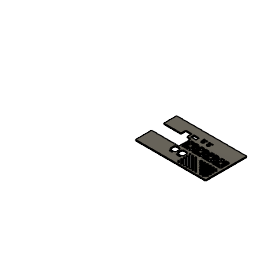
HomecurrentMoniter_Top Plate HCM UPDATED (Autodesk Fusion 360 design; units mm, degrees)
part number: 2026-06-16-14-02-59-231
Autodesk Fusion 360 part; units mm, degrees
(part 1 of 5)
sketch "Sketch1" plane through (0, 0, 20) normal (0, 0, 1) x (-1, 0, 0)
  line L0 (-199.377, 36.7921) -> (-199.377, 118.6521)
  line L1 (-199.377, 118.6521) -> (-338.527, 118.6521)
  line L2 (-338.527, 118.6521) -> (-338.527, 36.7921)
  line L3 (-338.527, 36.7921) -> (-199.377, 36.7921)
  line L4 (-257.2248, 89.2793) -> (-251.8248, 89.2793)
  arc A0 (-251.8248, 89.2793) -> (-248.7748, 92.3293) centre (-251.8248, 92.3293) ccw
  line L5 (-248.7748, 92.3293) -> (-248.7748, 97.7293)
  arc A1 (-248.7748, 97.7293) -> (-251.8248, 100.7793) centre (-251.8248, 97.7293) ccw
  line L6 (-251.8248, 100.7793) -> (-257.2248, 100.7793)
  arc A2 (-257.2248, 100.7793) -> (-260.2748, 97.7293) centre (-257.2248, 97.7293) ccw
  line L7 (-260.2748, 97.7293) -> (-260.2748, 92.3293)
  arc A3 (-260.2748, 92.3293) -> (-257.2248, 89.2793) centre (-257.2248, 92.3293) ccw
  line L8 (-271.6198, 89.1213) -> (-266.2198, 89.1213)
  arc A4 (-266.2198, 89.1213) -> (-263.1698, 92.1713) centre (-266.2198, 92.1713) ccw
  arc A5 (-274.6698, 92.1713) -> (-271.6198, 89.1213) centre (-271.6198, 92.1713) ccw
  line L9 (-274.6698, 97.5713) -> (-274.6698, 92.1713)
  arc A6 (-271.6198, 100.6213) -> (-274.6698, 97.5713) centre (-271.6198, 97.5713) ccw
  line L10 (-266.2198, 100.6213) -> (-271.6198, 100.6213)
  arc A7 (-263.1698, 97.5713) -> (-266.2198, 100.6213) centre (-266.2198, 97.5713) ccw
  line L11 (-263.1698, 92.1713) -> (-263.1698, 97.5713)
  arc A8 (-268.8911, 56.8718) -> (-268.8911, 54.5394) centre (-270.3911, 55.7056) ccw
  line L12 (-268.8911, 56.8718) -> (-268.8911, 54.5394)
  arc A9 (-280.0411, 56.9618) -> (-280.0411, 54.6294) centre (-281.5411, 55.7956) ccw
  line L13 (-280.0411, 56.9618) -> (-280.0411, 54.6294)
  line L14 (-251.0886, 55.7428) -> (-251.3426, 55.9968)
  line L15 (-251.3426, 55.9968) -> (-253.3746, 55.9968)
  line L16 (-253.3746, 55.9968) -> (-253.6286, 55.7428)
  line L17 (-253.6286, 55.7428) -> (-253.8826, 55.9968)
  line L18 (-253.8826, 55.9968) -> (-255.9146, 55.9968)
  line L19 (-255.9146, 55.9968) -> (-256.1686, 55.7428)
  line L20 (-256.1686, 55.7428) -> (-256.4226, 55.9968)
  line L21 (-256.4226, 55.9968) -> (-258.4546, 55.9968)
  line L22 (-258.4546, 55.9968) -> (-258.7086, 55.7428)
  line L23 (-258.7086, 55.7428) -> (-258.7086, 53.7108)
  line L24 (-258.7086, 53.7108) -> (-258.4546, 53.4568)
  line L25 (-258.4546, 53.4568) -> (-256.4226, 53.4568)
  line L26 (-256.4226, 53.4568) -> (-256.1686, 53.7108)
  line L27 (-256.1686, 53.7108) -> (-255.9146, 53.4568)
  line L28 (-255.9146, 53.4568) -> (-253.8826, 53.4568)
  line L29 (-253.8826, 53.4568) -> (-253.6286, 53.7108)
  line L30 (-253.6286, 53.7108) -> (-253.3746, 53.4568)
  line L31 (-253.3746, 53.4568) -> (-251.3426, 53.4568)
  line L32 (-251.3426, 53.4568) -> (-251.0886, 53.7108)
  line L33 (-251.0886, 53.7108) -> (-251.0886, 55.7428)
  line L34 (-234.5786, 55.7428) -> (-234.8326, 55.9968)
  line L35 (-234.8326, 55.9968) -> (-236.8646, 55.9968)
  line L36 (-236.8646, 55.9968) -> (-237.1186, 55.7428)
  line L37 (-237.1186, 55.7428) -> (-237.3726, 55.9968)
  line L38 (-237.3726, 55.9968) -> (-239.4046, 55.9968)
  line L39 (-239.4046, 55.9968) -> (-239.6586, 55.7428)
  line L40 (-239.6586, 55.7428) -> (-239.9126, 55.9968)
  line L41 (-239.9126, 55.9968) -> (-241.9446, 55.9968)
  line L42 (-241.9446, 55.9968) -> (-242.1986, 55.7428)
  line L43 (-242.1986, 55.7428) -> (-242.4526, 55.9968)
  line L44 (-242.4526, 55.9968) -> (-244.4846, 55.9968)
  line L45 (-244.4846, 55.9968) -> (-244.7386, 55.7428)
  line L46 (-244.7386, 55.7428) -> (-244.7386, 53.7108)
  line L47 (-244.7386, 53.7108) -> (-244.4846, 53.4568)
  line L48 (-244.4846, 53.4568) -> (-242.4526, 53.4568)
  line L49 (-242.4526, 53.4568) -> (-242.1986, 53.7108)
  line L50 (-242.1986, 53.7108) -> (-241.9446, 53.4568)
  line L51 (-241.9446, 53.4568) -> (-239.9126, 53.4568)
  line L52 (-239.9126, 53.4568) -> (-239.6586, 53.7108)
  line L53 (-239.6586, 53.7108) -> (-239.4046, 53.4568)
  line L54 (-239.4046, 53.4568) -> (-237.3726, 53.4568)
  line L55 (-237.3726, 53.4568) -> (-237.1186, 53.7108)
  line L56 (-237.1186, 53.7108) -> (-236.8646, 53.4568)
  line L57 (-236.8646, 53.4568) -> (-234.8326, 53.4568)
  line L58 (-234.8326, 53.4568) -> (-234.5786, 53.7108)
  line L59 (-234.5786, 53.7108) -> (-234.5786, 55.7428)
  line L60 (-249.9009, 53) -> (-259.9009, 53)
  line L61 (-259.9009, 53) -> (-259.9009, 59)
  line L62 (-259.9009, 59) -> (-249.9009, 59)
  line L63 (-249.9009, 59) -> (-249.9009, 53)
  line L64 (-233.633, 53) -> (-245.633, 53)
  line L65 (-245.633, 53) -> (-245.633, 75)
  line L66 (-245.633, 75) -> (-233.633, 75)
  line L67 (-233.633, 75) -> (-233.633, 53)
  circle A10 centre (-270.3911, 55.7056) radius 3
  circle A11 centre (-281.5411, 55.7956) radius 3
  line L68 (-232.1048, 83.5518) -> (-224.9198, 83.5518)
  line L69 (-224.9198, 83.5518) -> (-224.9198, 65.5518)
  line L70 (-224.9198, 65.5518) -> (-232.1048, 65.5518)
  line L71 (-232.1098, 65.5518) -> (-232.1048, 65.5518)
  line L72 (-232.2048, 65.5518) -> (-232.1098, 65.5518)
  arc A12 (-232.2048, 65.5518) -> (-232.7048, 65.5518) centre (-232.4548, 65.5518) ccw
  line L73 (-232.7098, 65.5518) -> (-232.7048, 65.5518)
  line L74 (-232.8048, 65.5518) -> (-232.7098, 65.5518)
  line L75 (-232.8048, 65.5518) -> (-233.3748, 65.5518)
  line L76 (-233.3798, 65.5518) -> (-233.3748, 65.5518)
  line L77 (-233.4748, 65.5518) -> (-233.3798, 65.5518)
  arc A13 (-233.4748, 65.5518) -> (-233.9748, 65.5518) centre (-233.7248, 65.5518) ccw
  line L78 (-233.9798, 65.5518) -> (-233.9748, 65.5518)
  line L79 (-234.0748, 65.5518) -> (-233.9798, 65.5518)
  line L80 (-234.0748, 65.5518) -> (-234.6448, 65.5518)
  line L81 (-234.6498, 65.5518) -> (-234.6448, 65.5518)
  line L82 (-234.7448, 65.5518) -> (-234.6498, 65.5518)
  arc A14 (-234.7448, 65.5518) -> (-235.2448, 65.5518) centre (-234.9948, 65.5518) ccw
  line L83 (-235.2498, 65.5518) -> (-235.2448, 65.5518)
  line L84 (-235.3448, 65.5518) -> (-235.2498, 65.5518)
  line L85 (-235.3448, 65.5518) -> (-235.9148, 65.5518)
  line L86 (-235.9198, 65.5518) -> (-235.9148, 65.5518)
  line L87 (-236.0148, 65.5518) -> (-235.9198, 65.5518)
  arc A15 (-236.0148, 65.5518) -> (-236.5148, 65.5518) centre (-236.2648, 65.5518) ccw
  line L88 (-236.5198, 65.5518) -> (-236.5148, 65.5518)
  line L89 (-236.6148, 65.5518) -> (-236.5198, 65.5518)
  line L90 (-236.6148, 65.5518) -> (-237.1848, 65.5518)
  line L91 (-237.1898, 65.5518) -> (-237.1848, 65.5518)
  line L92 (-237.2848, 65.5518) -> (-237.1898, 65.5518)
  arc A16 (-237.2848, 65.5518) -> (-237.7848, 65.5518) centre (-237.5348, 65.5518) ccw
  line L93 (-237.7898, 65.5518) -> (-237.7848, 65.5518)
  line L94 (-237.8848, 65.5518) -> (-237.7898, 65.5518)
  line L95 (-237.8848, 65.5518) -> (-238.4548, 65.5518)
  line L96 (-238.4598, 65.5518) -> (-238.4548, 65.5518)
  line L97 (-238.5548, 65.5518) -> (-238.4598, 65.5518)
  arc A17 (-238.5548, 65.5518) -> (-239.0548, 65.5518) centre (-238.8048, 65.5518) ccw
  line L98 (-239.0598, 65.5518) -> (-239.0548, 65.5518)
  line L99 (-239.1548, 65.5518) -> (-239.0598, 65.5518)
  line L100 (-239.1548, 65.5518) -> (-239.7248, 65.5518)
  line L101 (-239.7298, 65.5518) -> (-239.7248, 65.5518)
  line L102 (-239.8248, 65.5518) -> (-239.7298, 65.5518)
  arc A18 (-239.8248, 65.5518) -> (-240.3248, 65.5518) centre (-240.0748, 65.5518) ccw
  line L103 (-240.3298, 65.5518) -> (-240.3248, 65.5518)
  line L104 (-240.4248, 65.5518) -> (-240.3298, 65.5518)
  line L105 (-240.4248, 65.5518) -> (-240.9948, 65.5518)
  line L106 (-240.9998, 65.5518) -> (-240.9948, 65.5518)
  line L107 (-241.0948, 65.5518) -> (-240.9998, 65.5518)
  arc A19 (-241.0948, 65.5518) -> (-241.5948, 65.5518) centre (-241.3448, 65.5518) ccw
  line L108 (-241.5998, 65.5518) -> (-241.5948, 65.5518)
  line L109 (-241.6948, 65.5518) -> (-241.5998, 65.5518)
  line L110 (-241.6948, 65.5518) -> (-242.2648, 65.5518)
  line L111 (-242.2698, 65.5518) -> (-242.2648, 65.5518)
  line L112 (-242.3648, 65.5518) -> (-242.2698, 65.5518)
  arc A20 (-242.3648, 65.5518) -> (-242.8648, 65.5518) centre (-242.6148, 65.5518) ccw
  line L113 (-242.8698, 65.5518) -> (-242.8648, 65.5518)
  line L114 (-242.9648, 65.5518) -> (-242.8698, 65.5518)
  line L115 (-242.9648, 65.5518) -> (-243.5348, 65.5518)
  line L116 (-243.5398, 65.5518) -> (-243.5348, 65.5518)
  line L117 (-243.6348, 65.5518) -> (-243.5398, 65.5518)
  arc A21 (-243.6348, 65.5518) -> (-244.1348, 65.5518) centre (-243.8848, 65.5518) ccw
  line L118 (-244.1398, 65.5518) -> (-244.1348, 65.5518)
  line L119 (-244.2348, 65.5518) -> (-244.1398, 65.5518)
  line L120 (-244.2348, 65.5518) -> (-244.8048, 65.5518)
  line L121 (-244.8098, 65.5518) -> (-244.8048, 65.5518)
  line L122 (-244.9048, 65.5518) -> (-244.8098, 65.5518)
  arc A22 (-244.9048, 65.5518) -> (-245.4048, 65.5518) centre (-245.1548, 65.5518) ccw
  line L123 (-245.4098, 65.5518) -> (-245.4048, 65.5518)
  line L124 (-245.5048, 65.5518) -> (-245.4098, 65.5518)
  line L125 (-245.5048, 65.5518) -> (-246.0748, 65.5518)
  line L126 (-246.0798, 65.5518) -> (-246.0748, 65.5518)
  line L127 (-246.1748, 65.5518) -> (-246.0798, 65.5518)
  arc A23 (-246.1748, 65.5518) -> (-246.6748, 65.5518) centre (-246.4248, 65.5518) ccw
  line L128 (-246.6798, 65.5518) -> (-246.6748, 65.5518)
  line L129 (-246.7748, 65.5518) -> (-246.6798, 65.5518)
  line L130 (-246.7748, 65.5518) -> (-247.3448, 65.5518)
  line L131 (-247.3498, 65.5518) -> (-247.3448, 65.5518)
  line L132 (-247.4448, 65.5518) -> (-247.3498, 65.5518)
  arc A24 (-247.4448, 65.5518) -> (-247.9448, 65.5518) centre (-247.6948, 65.5518) ccw
  line L133 (-247.9498, 65.5518) -> (-247.9448, 65.5518)
  line L134 (-248.0448, 65.5518) -> (-247.9498, 65.5518)
  line L135 (-248.0448, 65.5518) -> (-248.6148, 65.5518)
  line L136 (-248.6198, 65.5518) -> (-248.6148, 65.5518)
  line L137 (-248.7148, 65.5518) -> (-248.6198, 65.5518)
  arc A25 (-248.7148, 65.5518) -> (-249.2148, 65.5518) centre (-248.9648, 65.5518) ccw
  line L138 (-249.2198, 65.5518) -> (-249.2148, 65.5518)
  line L139 (-249.3148, 65.5518) -> (-249.2198, 65.5518)
  line L140 (-249.3148, 65.5518) -> (-250.4198, 65.5518)
  line L141 (-250.4198, 65.5518) -> (-250.4198, 68.4418)
  line L142 (-250.4198, 68.5369) -> (-250.4198, 68.4418)
  line L143 (-250.4198, 68.5418) -> (-250.4198, 68.5369)
  arc A26 (-250.4198, 68.5418) -> (-250.4198, 69.0418) centre (-250.4198, 68.7918) ccw
  line L144 (-250.4198, 69.1368) -> (-250.4198, 69.0418)
  line L145 (-250.4198, 69.1418) -> (-250.4198, 69.1368)
  line L146 (-250.4198, 69.1418) -> (-250.4198, 69.7118)
  line L147 (-250.4198, 69.8069) -> (-250.4198, 69.7118)
  line L148 (-250.4198, 69.8118) -> (-250.4198, 69.8069)
  arc A27 (-250.4198, 69.8118) -> (-250.4198, 70.3118) centre (-250.4198, 70.0618) ccw
  line L149 (-250.4198, 70.4068) -> (-250.4198, 70.3118)
  line L150 (-250.4198, 70.4118) -> (-250.4198, 70.4068)
  line L151 (-250.4198, 70.4118) -> (-250.4198, 70.9818)
  line L152 (-250.4198, 71.0769) -> (-250.4198, 70.9818)
  line L153 (-250.4198, 71.0818) -> (-250.4198, 71.0769)
  arc A28 (-250.4198, 71.0818) -> (-250.4198, 71.5818) centre (-250.4198, 71.3318) ccw
  line L154 (-250.4198, 71.6768) -> (-250.4198, 71.5818)
  line L155 (-250.4198, 71.6818) -> (-250.4198, 71.6768)
  line L156 (-250.4198, 71.6818) -> (-250.4198, 72.2518)
  line L157 (-250.4198, 72.3469) -> (-250.4198, 72.2518)
  line L158 (-250.4198, 72.3518) -> (-250.4198, 72.3469)
  arc A29 (-250.4198, 72.3518) -> (-250.4198, 72.8518) centre (-250.4198, 72.6018) ccw
  line L159 (-250.4198, 72.9468) -> (-250.4198, 72.8518)
  line L160 (-250.4198, 72.9518) -> (-250.4198, 72.9468)
  line L161 (-250.4198, 72.9518) -> (-250.4198, 73.5218)
  line L162 (-250.4198, 73.6169) -> (-250.4198, 73.5218)
  line L163 (-250.4198, 73.6218) -> (-250.4198, 73.6169)
  arc A30 (-250.4198, 73.6218) -> (-250.4198, 74.1218) centre (-250.4198, 73.8718) ccw
  line L164 (-250.4198, 74.2168) -> (-250.4198, 74.1218)
  line L165 (-250.4198, 74.2218) -> (-250.4198, 74.2168)
  line L166 (-250.4198, 74.2218) -> (-250.4198, 74.7918)
  line L167 (-250.4198, 74.8869) -> (-250.4198, 74.7918)
  line L168 (-250.4198, 74.8918) -> (-250.4198, 74.8869)
  arc A31 (-250.4198, 74.8918) -> (-250.4198, 75.3918) centre (-250.4198, 75.1418) ccw
  line L169 (-250.4198, 75.4868) -> (-250.4198, 75.3918)
  line L170 (-250.4198, 75.4918) -> (-250.4198, 75.4868)
  line L171 (-250.4198, 75.4918) -> (-250.4198, 76.0618)
  line L172 (-250.4198, 76.1569) -> (-250.4198, 76.0618)
  line L173 (-250.4198, 76.1618) -> (-250.4198, 76.1569)
  arc A32 (-250.4198, 76.1618) -> (-250.4198, 76.6618) centre (-250.4198, 76.4118) ccw
  line L174 (-250.4198, 76.7568) -> (-250.4198, 76.6618)
  line L175 (-250.4198, 76.7618) -> (-250.4198, 76.7568)
  line L176 (-250.4198, 76.7618) -> (-250.4198, 77.3318)
  line L177 (-250.4198, 77.4269) -> (-250.4198, 77.3318)
  line L178 (-250.4198, 77.4318) -> (-250.4198, 77.4269)
  arc A33 (-250.4198, 77.4318) -> (-250.4198, 77.9318) centre (-250.4198, 77.6818) ccw
  line L179 (-250.4198, 78.0268) -> (-250.4198, 77.9318)
  line L180 (-250.4198, 78.0318) -> (-250.4198, 78.0268)
  line L181 (-250.4198, 78.0318) -> (-250.4198, 78.6018)
  line L182 (-250.4198, 78.6969) -> (-250.4198, 78.6018)
  line L183 (-250.4198, 78.7018) -> (-250.4198, 78.6969)
  arc A34 (-250.4198, 78.7018) -> (-250.4198, 79.2018) centre (-250.4198, 78.9518) ccw
  line L184 (-250.4198, 79.2968) -> (-250.4198, 79.2018)
  line L185 (-250.4198, 79.3018) -> (-250.4198, 79.2968)
  line L186 (-250.4198, 79.3018) -> (-250.4198, 79.8718)
  line L187 (-250.4198, 79.9669) -> (-250.4198, 79.8718)
  line L188 (-250.4198, 79.9718) -> (-250.4198, 79.9669)
  arc A35 (-250.4198, 79.9718) -> (-250.4198, 80.4718) centre (-250.4198, 80.2218) ccw
  line L189 (-250.4198, 80.5668) -> (-250.4198, 80.4718)
  line L190 (-250.4198, 80.5718) -> (-250.4198, 80.5668)
  line L191 (-250.4198, 80.5718) -> (-250.4198, 83.5518)
  line L192 (-250.4198, 83.5518) -> (-249.3148, 83.5518)
  line L193 (-249.2198, 83.5518) -> (-249.3148, 83.5518)
  line L194 (-249.2148, 83.5518) -> (-249.2198, 83.5518)
  arc A36 (-249.2148, 83.5518) -> (-248.7148, 83.5518) centre (-248.9648, 83.5518) ccw
  line L195 (-248.6198, 83.5518) -> (-248.7148, 83.5518)
  line L196 (-248.6148, 83.5518) -> (-248.6198, 83.5518)
  line L197 (-248.6148, 83.5518) -> (-248.0448, 83.5518)
  line L198 (-247.9498, 83.5518) -> (-248.0448, 83.5518)
  line L199 (-247.9448, 83.5518) -> (-247.9498, 83.5518)
  arc A37 (-247.9448, 83.5518) -> (-247.4448, 83.5518) centre (-247.6948, 83.5518) ccw
  line L200 (-247.3498, 83.5518) -> (-247.4448, 83.5518)
  line L201 (-247.3448, 83.5518) -> (-247.3498, 83.5518)
  line L202 (-247.3448, 83.5518) -> (-246.7748, 83.5518)
  line L203 (-246.6798, 83.5518) -> (-246.7748, 83.5518)
  line L204 (-246.6748, 83.5518) -> (-246.6798, 83.5518)
  arc A38 (-246.6748, 83.5518) -> (-246.1748, 83.5518) centre (-246.4248, 83.5518) ccw
  line L205 (-246.0798, 83.5518) -> (-246.1748, 83.5518)
  line L206 (-246.0748, 83.5518) -> (-246.0798, 83.5518)
  line L207 (-246.0748, 83.5518) -> (-245.5048, 83.5518)
  line L208 (-245.4098, 83.5518) -> (-245.5048, 83.5518)
  line L209 (-245.4048, 83.5518) -> (-245.4098, 83.5518)
  arc A39 (-245.4048, 83.5518) -> (-244.9048, 83.5518) centre (-245.1548, 83.5518) ccw
  line L210 (-244.8098, 83.5518) -> (-244.9048, 83.5518)
  line L211 (-244.8048, 83.5518) -> (-244.8098, 83.5518)
  line L212 (-244.8048, 83.5518) -> (-244.2348, 83.5518)
  line L213 (-244.1398, 83.5518) -> (-244.2348, 83.5518)
  line L214 (-244.1348, 83.5518) -> (-244.1398, 83.5518)
  arc A40 (-244.1348, 83.5518) -> (-243.6348, 83.5518) centre (-243.8848, 83.5518) ccw
  line L215 (-243.5398, 83.5518) -> (-243.6348, 83.5518)
  line L216 (-243.5348, 83.5518) -> (-243.5398, 83.5518)
  line L217 (-243.5348, 83.5518) -> (-242.9648, 83.5518)
  line L218 (-242.8698, 83.5518) -> (-242.9648, 83.5518)
  line L219 (-242.8648, 83.5518) -> (-242.8698, 83.5518)
  arc A41 (-242.8648, 83.5518) -> (-242.3648, 83.5518) centre (-242.6148, 83.5518) ccw
  line L220 (-242.2698, 83.5518) -> (-242.3648, 83.5518)
  line L221 (-242.2648, 83.5518) -> (-242.2698, 83.5518)
  line L222 (-242.2648, 83.5518) -> (-241.6948, 83.5518)
  line L223 (-241.6148, 83.5518) -> (-241.6948, 83.5518)
  line L224 (-241.5998, 83.5518) -> (-241.6148, 83.5518)
  line L225 (-241.5948, 83.5518) -> (-241.5998, 83.5518)
  line L226 (-241.5148, 83.5518) -> (-241.5948, 83.5518)
  arc A42 (-241.5148, 83.5518) -> (-241.3048, 83.305) centre (-241.2648, 83.5518) ccw
  arc A43 (-241.3048, 83.305) -> (-241.0948, 83.5518) centre (-241.3448, 83.5518) ccw
  line L227 (-241.0148, 83.5518) -> (-241.0948, 83.5518)
  line L228 (-240.9998, 83.5518) -> (-241.0148, 83.5518)
  line L229 (-240.9948, 83.5518) -> (-240.9998, 83.5518)
  line L230 (-240.9148, 83.5518) -> (-240.9948, 83.5518)
  line L231 (-240.9148, 83.5518) -> (-240.4248, 83.5518)
  line L232 (-240.3298, 83.5518) -> (-240.4248, 83.5518)
  line L233 (-240.3248, 83.5518) -> (-240.3298, 83.5518)
  arc A44 (-240.3248, 83.5518) -> (-239.8248, 83.5518) centre (-240.0748, 83.5518) ccw
  line L234 (-239.7298, 83.5518) -> (-239.8248, 83.5518)
  line L235 (-239.7248, 83.5518) -> (-239.7298, 83.5518)
  line L236 (-239.7248, 83.5518) -> (-239.1548, 83.5518)
  line L237 (-239.0598, 83.5518) -> (-239.1548, 83.5518)
  line L238 (-239.0548, 83.5518) -> (-239.0598, 83.5518)
  arc A45 (-239.0548, 83.5518) -> (-238.5548, 83.5518) centre (-238.8048, 83.5518) ccw
  line L239 (-238.4598, 83.5518) -> (-238.5548, 83.5518)
  line L240 (-238.4548, 83.5518) -> (-238.4598, 83.5518)
  line L241 (-238.4548, 83.5518) -> (-237.8848, 83.5518)
  line L242 (-237.7898, 83.5518) -> (-237.8848, 83.5518)
  line L243 (-237.7848, 83.5518) -> (-237.7898, 83.5518)
  arc A46 (-237.7848, 83.5518) -> (-237.2848, 83.5518) centre (-237.5348, 83.5518) ccw
  line L244 (-237.1898, 83.5518) -> (-237.2848, 83.5518)
  line L245 (-237.1848, 83.5518) -> (-237.1898, 83.5518)
  line L246 (-237.1848, 83.5518) -> (-236.6148, 83.5518)
  line L247 (-236.5198, 83.5518) -> (-236.6148, 83.5518)
  line L248 (-236.5148, 83.5518) -> (-236.5198, 83.5518)
  arc A47 (-236.5148, 83.5518) -> (-236.0148, 83.5518) centre (-236.2648, 83.5518) ccw
  line L249 (-235.9198, 83.5518) -> (-236.0148, 83.5518)
  line L250 (-235.9148, 83.5518) -> (-235.9198, 83.5518)
  line L251 (-235.9148, 83.5518) -> (-235.3448, 83.5518)
  line L252 (-235.2498, 83.5518) -> (-235.3448, 83.5518)
  line L253 (-235.2448, 83.5518) -> (-235.2498, 83.5518)
  arc A48 (-235.2448, 83.5518) -> (-234.7448, 83.5518) centre (-234.9948, 83.5518) ccw
  line L254 (-234.6498, 83.5518) -> (-234.7448, 83.5518)
  line L255 (-234.6448, 83.5518) -> (-234.6498, 83.5518)
  line L256 (-234.6448, 83.5518) -> (-234.0748, 83.5518)
  line L257 (-233.9798, 83.5518) -> (-234.0748, 83.5518)
  line L258 (-233.9748, 83.5518) -> (-233.9798, 83.5518)
  arc A49 (-233.9748, 83.5518) -> (-233.4748, 83.5518) centre (-233.7248, 83.5518) ccw
  line L259 (-233.3798, 83.5518) -> (-233.4748, 83.5518)
  line L260 (-233.3748, 83.5518) -> (-233.3798, 83.5518)
  line L261 (-233.3748, 83.5518) -> (-232.8048, 83.5518)
  line L262 (-232.7098, 83.5518) -> (-232.8048, 83.5518)
  line L263 (-232.7048, 83.5518) -> (-232.7098, 83.5518)
  arc A50 (-232.7048, 83.5518) -> (-232.2048, 83.5518) centre (-232.4548, 83.5518) ccw
  line L264 (-232.1098, 83.5518) -> (-232.2048, 83.5518)
  line L265 (-232.1048, 83.5518) -> (-232.1098, 83.5518)
  line L266 (-232.1098, 62.5518) -> (-232.1048, 62.5518)
  line L267 (-221.9198, 62.5518) -> (-232.1048, 62.5518)
  line L268 (-232.1048, 86.5518) -> (-221.9198, 86.5518)
  line L269 (-232.1048, 86.5518) -> (-232.1098, 86.5518)
  line L270 (-232.1098, 86.5518) -> (-232.2048, 86.5518)
  arc A51 (-232.2048, 86.5518) -> (-232.4548, 86.5414) centre (-232.2048, 83.5518) ccw
  arc A52 (-232.4548, 86.5414) -> (-232.7048, 86.5518) centre (-232.7048, 83.5518) ccw
  line L271 (-232.7048, 86.5518) -> (-232.7098, 86.5518)
  line L272 (-232.7098, 86.5518) -> (-232.8048, 86.5518)
  line L273 (-233.3748, 86.5518) -> (-232.8048, 86.5518)
  line L274 (-233.3748, 86.5518) -> (-233.3798, 86.5518)
  line L275 (-233.3798, 86.5518) -> (-233.4748, 86.5518)
  arc A53 (-233.4748, 86.5518) -> (-233.7248, 86.5414) centre (-233.4748, 83.5518) ccw
  arc A54 (-233.7248, 86.5414) -> (-233.9748, 86.5518) centre (-233.9748, 83.5518) ccw
  line L276 (-233.9748, 86.5518) -> (-233.9798, 86.5518)
  line L277 (-233.9798, 86.5518) -> (-234.0748, 86.5518)
  line L278 (-234.6448, 86.5518) -> (-234.0748, 86.5518)
  line L279 (-234.6448, 86.5518) -> (-234.6498, 86.5518)
  line L280 (-234.6498, 86.5518) -> (-234.7448, 86.5518)
  arc A55 (-234.7448, 86.5518) -> (-234.9948, 86.5414) centre (-234.7448, 83.5518) ccw
  arc A56 (-234.9948, 86.5414) -> (-235.2448, 86.5518) centre (-235.2448, 83.5518) ccw
  line L281 (-235.2448, 86.5518) -> (-235.2498, 86.5518)
  line L282 (-235.2498, 86.5518) -> (-235.3448, 86.5518)
  line L283 (-235.9148, 86.5518) -> (-235.3448, 86.5518)
  line L284 (-235.9148, 86.5518) -> (-235.9198, 86.5518)
  line L285 (-235.9198, 86.5518) -> (-236.0148, 86.5518)
  arc A57 (-236.0148, 86.5518) -> (-236.2648, 86.5414) centre (-236.0148, 83.5518) ccw
  arc A58 (-236.2648, 86.5414) -> (-236.5148, 86.5518) centre (-236.5148, 83.5518) ccw
  line L286 (-236.5148, 86.5518) -> (-236.5198, 86.5518)
  line L287 (-236.5198, 86.5518) -> (-236.6148, 86.5518)
  line L288 (-237.1848, 86.5518) -> (-236.6148, 86.5518)
  line L289 (-237.1848, 86.5518) -> (-237.1898, 86.5518)
  line L290 (-237.1898, 86.5518) -> (-237.2848, 86.5518)
  arc A59 (-237.2848, 86.5518) -> (-237.5348, 86.5414) centre (-237.2848, 83.5518) ccw
  arc A60 (-237.5348, 86.5414) -> (-237.7848, 86.5518) centre (-237.7848, 83.5518) ccw
  line L291 (-237.7848, 86.5518) -> (-237.7898, 86.5518)
  line L292 (-237.7898, 86.5518) -> (-237.8848, 86.5518)
  line L293 (-238.4548, 86.5518) -> (-237.8848, 86.5518)
  line L294 (-238.4548, 86.5518) -> (-238.4598, 86.5518)
  line L295 (-238.4598, 86.5518) -> (-238.5548, 86.5518)
  arc A61 (-238.5548, 86.5518) -> (-238.8048, 86.5414) centre (-238.5548, 83.5518) ccw
  arc A62 (-238.8048, 86.5414) -> (-239.0548, 86.5518) centre (-239.0548, 83.5518) ccw
  line L296 (-239.0548, 86.5518) -> (-239.0598, 86.5518)
  line L297 (-239.0598, 86.5518) -> (-239.1548, 86.5518)
  line L298 (-239.7248, 86.5518) -> (-239.1548, 86.5518)
  line L299 (-239.7248, 86.5518) -> (-239.7298, 86.5518)
  line L300 (-239.7298, 86.5518) -> (-239.8248, 86.5518)
  arc A63 (-239.8248, 86.5518) -> (-240.0748, 86.5414) centre (-239.8248, 83.5518) ccw
  arc A64 (-240.0748, 86.5414) -> (-240.3248, 86.5518) centre (-240.3248, 83.5518) ccw
  line L301 (-240.3248, 86.5518) -> (-240.3298, 86.5518)
  line L302 (-240.3298, 86.5518) -> (-240.4248, 86.5518)
  line L303 (-240.9148, 86.5518) -> (-240.4248, 86.5518)
  line L304 (-240.9148, 86.5518) -> (-240.9948, 86.5518)
  line L305 (-240.9948, 86.5518) -> (-240.9998, 86.5518)
  line L306 (-240.9998, 86.5518) -> (-241.0148, 86.5518)
  line L307 (-241.0148, 86.5518) -> (-241.0948, 86.5518)
  arc A65 (-241.0948, 86.5518) -> (-241.3048, 86.5445) centre (-241.0948, 83.5518) ccw
  arc A66 (-241.3048, 86.5445) -> (-241.5148, 86.5518) centre (-241.5148, 83.5518) ccw
  line L308 (-241.5148, 86.5518) -> (-241.5948, 86.5518)
  line L309 (-241.5948, 86.5518) -> (-241.5998, 86.5518)
  line L310 (-241.5998, 86.5518) -> (-241.6148, 86.5518)
  line L311 (-241.6148, 86.5518) -> (-241.6948, 86.5518)
  line L312 (-242.2648, 86.5518) -> (-241.6948, 86.5518)
  line L313 (-242.2648, 86.5518) -> (-242.2698, 86.5518)
  line L314 (-242.2698, 86.5518) -> (-242.3648, 86.5518)
  arc A67 (-242.3648, 86.5518) -> (-242.6148, 86.5414) centre (-242.3648, 83.5518) ccw
  arc A68 (-242.6148, 86.5414) -> (-242.8648, 86.5518) centre (-242.8648, 83.5518) ccw
  line L315 (-242.8648, 86.5518) -> (-242.8698, 86.5518)
  line L316 (-242.8698, 86.5518) -> (-242.9648, 86.5518)
  line L317 (-243.5348, 86.5518) -> (-242.9648, 86.5518)
  line L318 (-243.5348, 86.5518) -> (-243.5398, 86.5518)
  line L319 (-243.5398, 86.5518) -> (-243.6348, 86.5518)
  arc A69 (-243.6348, 86.5518) -> (-243.8848, 86.5414) centre (-243.6348, 83.5518) ccw
  arc A70 (-243.8848, 86.5414) -> (-244.1348, 86.5518) centre (-244.1348, 83.5518) ccw
  line L320 (-244.1348, 86.5518) -> (-244.1398, 86.5518)
  line L321 (-244.1398, 86.5518) -> (-244.2348, 86.5518)
  line L322 (-244.8048, 86.5518) -> (-244.2348, 86.5518)
  line L323 (-244.8048, 86.5518) -> (-244.8098, 86.5518)
  line L324 (-244.8098, 86.5518) -> (-244.9048, 86.5518)
  arc A71 (-244.9048, 86.5518) -> (-245.1548, 86.5414) centre (-244.9048, 83.5518) ccw
  arc A72 (-245.1548, 86.5414) -> (-245.4048, 86.5518) centre (-245.4048, 83.5518) ccw
  line L325 (-245.4048, 86.5518) -> (-245.4098, 86.5518)
  line L326 (-245.4098, 86.5518) -> (-245.5048, 86.5518)
  line L327 (-246.0748, 86.5518) -> (-245.5048, 86.5518)
  line L328 (-246.0748, 86.5518) -> (-246.0798, 86.5518)
  line L329 (-246.0798, 86.5518) -> (-246.1748, 86.5518)
  arc A73 (-246.1748, 86.5518) -> (-246.4248, 86.5414) centre (-246.1748, 83.5518) ccw
  arc A74 (-246.4248, 86.5414) -> (-246.6748, 86.5518) centre (-246.6748, 83.5518) ccw
  line L330 (-246.6748, 86.5518) -> (-246.6798, 86.5518)
  line L331 (-246.6798, 86.5518) -> (-246.7748, 86.5518)
  line L332 (-247.3448, 86.5518) -> (-246.7748, 86.5518)
  line L333 (-247.3448, 86.5518) -> (-247.3498, 86.5518)
  line L334 (-247.3498, 86.5518) -> (-247.4448, 86.5518)
  arc A75 (-247.4448, 86.5518) -> (-247.6948, 86.5414) centre (-247.4448, 83.5518) ccw
  arc A76 (-247.6948, 86.5414) -> (-247.9448, 86.5518) centre (-247.9448, 83.5518) ccw
  line L335 (-247.9448, 86.5518) -> (-247.9498, 86.5518)
  line L336 (-247.9498, 86.5518) -> (-248.0448, 86.5518)
  line L337 (-248.6148, 86.5518) -> (-248.0448, 86.5518)
  line L338 (-248.6148, 86.5518) -> (-248.6198, 86.5518)
  line L339 (-248.6198, 86.5518) -> (-248.7148, 86.5518)
  arc A77 (-248.7148, 86.5518) -> (-248.9648, 86.5414) centre (-248.7148, 83.5518) ccw
  arc A78 (-248.9648, 86.5414) -> (-249.2148, 86.5518) centre (-249.2148, 83.5518) ccw
  line L340 (-249.2148, 86.5518) -> (-249.2198, 86.5518)
  line L341 (-249.2198, 86.5518) -> (-249.3148, 86.5518)
  line L342 (-252.4198, 86.5518) -> (-249.3148, 86.5518)
  line L343 (-253.4198, 80.5718) -> (-253.4198, 85.5518)
  line L344 (-253.4198, 80.5718) -> (-253.4198, 80.5668)
  line L345 (-253.4198, 80.5668) -> (-253.4198, 80.4718)
  arc A79 (-253.4198, 80.4718) -> (-253.4094, 80.2218) centre (-250.4198, 80.4718) ccw
  arc A80 (-253.4094, 80.2218) -> (-253.4198, 79.9718) centre (-250.4198, 79.9718) ccw
  line L346 (-253.4198, 79.9718) -> (-253.4198, 79.9669)
  line L347 (-253.4198, 79.9669) -> (-253.4198, 79.8718)
  line L348 (-253.4198, 79.3018) -> (-253.4198, 79.8718)
  line L349 (-253.4198, 79.3018) -> (-253.4198, 79.2968)
  line L350 (-253.4198, 79.2968) -> (-253.4198, 79.2018)
  arc A81 (-253.4198, 79.2018) -> (-253.4094, 78.9518) centre (-250.4198, 79.2018) ccw
  arc A82 (-253.4094, 78.9518) -> (-253.4198, 78.7018) centre (-250.4198, 78.7018) ccw
  line L351 (-253.4198, 78.7018) -> (-253.4198, 78.6969)
  line L352 (-253.4198, 78.6969) -> (-253.4198, 78.6018)
  line L353 (-253.4198, 78.0318) -> (-253.4198, 78.6018)
  line L354 (-253.4198, 78.0318) -> (-253.4198, 78.0268)
  line L355 (-253.4198, 78.0268) -> (-253.4198, 77.9318)
  arc A83 (-253.4198, 77.9318) -> (-253.4094, 77.6818) centre (-250.4198, 77.9318) ccw
  arc A84 (-253.4094, 77.6818) -> (-253.4198, 77.4318) centre (-250.4198, 77.4318) ccw
  line L356 (-253.4198, 77.4318) -> (-253.4198, 77.4269)
  line L357 (-253.4198, 77.4269) -> (-253.4198, 77.3318)
  line L358 (-253.4198, 76.7618) -> (-253.4198, 77.3318)
  line L359 (-253.4198, 76.7618) -> (-253.4198, 76.7568)
  line L360 (-253.4198, 76.7568) -> (-253.4198, 76.6618)
  arc A85 (-253.4198, 76.6618) -> (-253.4094, 76.4118) centre (-250.4198, 76.6618) ccw
  arc A86 (-253.4094, 76.4118) -> (-253.4198, 76.1618) centre (-250.4198, 76.1618) ccw
  line L361 (-253.4198, 76.1618) -> (-253.4198, 76.1569)
  line L362 (-253.4198, 76.1569) -> (-253.4198, 76.0618)
  line L363 (-253.4198, 75.4918) -> (-253.4198, 76.0618)
  line L364 (-253.4198, 75.4918) -> (-253.4198, 75.4868)
  line L365 (-253.4198, 75.4868) -> (-253.4198, 75.3918)
  arc A87 (-253.4198, 75.3918) -> (-253.4094, 75.1418) centre (-250.4198, 75.3918) ccw
  arc A88 (-253.4094, 75.1418) -> (-253.4198, 74.8918) centre (-250.4198, 74.8918) ccw
  line L366 (-253.4198, 74.8918) -> (-253.4198, 74.8869)
  line L367 (-253.4198, 74.8869) -> (-253.4198, 74.7918)
  line L368 (-253.4198, 74.2218) -> (-253.4198, 74.7918)
  line L369 (-253.4198, 74.2218) -> (-253.4198, 74.2168)
  line L370 (-253.4198, 74.2168) -> (-253.4198, 74.1218)
  arc A89 (-253.4198, 74.1218) -> (-253.4094, 73.8718) centre (-250.4198, 74.1218) ccw
  arc A90 (-253.4094, 73.8718) -> (-253.4198, 73.6218) centre (-250.4198, 73.6218) ccw
  line L371 (-253.4198, 73.6218) -> (-253.4198, 73.6169)
  line L372 (-253.4198, 73.6169) -> (-253.4198, 73.5218)
  line L373 (-253.4198, 72.9518) -> (-253.4198, 73.5218)
  line L374 (-253.4198, 72.9518) -> (-253.4198, 72.9468)
  line L375 (-253.4198, 72.9468) -> (-253.4198, 72.8518)
  arc A91 (-253.4198, 72.8518) -> (-253.4094, 72.6018) centre (-250.4198, 72.8518) ccw
  arc A92 (-253.4094, 72.6018) -> (-253.4198, 72.3518) centre (-250.4198, 72.3518) ccw
  line L376 (-253.4198, 72.3518) -> (-253.4198, 72.3469)
  line L377 (-253.4198, 72.3469) -> (-253.4198, 72.2518)
  line L378 (-253.4198, 71.6818) -> (-253.4198, 72.2518)
  line L379 (-253.4198, 71.6818) -> (-253.4198, 71.6768)
  line L380 (-253.4198, 71.6768) -> (-253.4198, 71.5818)
  arc A93 (-253.4198, 71.5818) -> (-253.4094, 71.3318) centre (-250.4198, 71.5818) ccw
  arc A94 (-253.4094, 71.3318) -> (-253.4198, 71.0818) centre (-250.4198, 71.0818) ccw
  line L381 (-253.4198, 71.0818) -> (-253.4198, 71.0769)
  line L382 (-253.4198, 71.0769) -> (-253.4198, 70.9818)
  line L383 (-253.4198, 70.4118) -> (-253.4198, 70.9818)
  line L384 (-253.4198, 70.4118) -> (-253.4198, 70.4068)
  line L385 (-253.4198, 70.4068) -> (-253.4198, 70.3118)
  arc A95 (-253.4198, 70.3118) -> (-253.4094, 70.0618) centre (-250.4198, 70.3118) ccw
  arc A96 (-253.4094, 70.0618) -> (-253.4198, 69.8118) centre (-250.4198, 69.8118) ccw
  line L386 (-253.4198, 69.8118) -> (-253.4198, 69.8069)
  line L387 (-253.4198, 69.8069) -> (-253.4198, 69.7118)
  line L388 (-253.4198, 69.1418) -> (-253.4198, 69.7118)
  line L389 (-253.4198, 69.1418) -> (-253.4198, 69.1368)
  line L390 (-253.4198, 69.1368) -> (-253.4198, 69.0418)
  arc A97 (-253.4198, 69.0418) -> (-253.4094, 68.7918) centre (-250.4198, 69.0418) ccw
  arc A98 (-253.4094, 68.7918) -> (-253.4198, 68.5418) centre (-250.4198, 68.5418) ccw
  line L391 (-253.4198, 68.5418) -> (-253.4198, 68.5369)
  line L392 (-253.4198, 68.5369) -> (-253.4198, 68.4418)
  line L393 (-253.4198, 63.5518) -> (-253.4198, 68.4418)
  line L394 (-249.3148, 62.5518) -> (-252.4198, 62.5518)
  line L395 (-249.3148, 62.5518) -> (-249.2198, 62.5518)
  line L396 (-249.2198, 62.5518) -> (-249.2148, 62.5518)
  arc A99 (-249.2148, 62.5518) -> (-248.9648, 62.5622) centre (-249.2148, 65.5518) ccw
  arc A100 (-248.9648, 62.5622) -> (-248.7148, 62.5518) centre (-248.7148, 65.5518) ccw
  line L397 (-248.7148, 62.5518) -> (-248.6198, 62.5518)
  line L398 (-248.6198, 62.5518) -> (-248.6148, 62.5518)
  line L399 (-248.0448, 62.5518) -> (-248.6148, 62.5518)
  line L400 (-248.0448, 62.5518) -> (-247.9498, 62.5518)
  line L401 (-247.9498, 62.5518) -> (-247.9448, 62.5518)
  arc A101 (-247.9448, 62.5518) -> (-247.6948, 62.5622) centre (-247.9448, 65.5518) ccw
  arc A102 (-247.6948, 62.5622) -> (-247.4448, 62.5518) centre (-247.4448, 65.5518) ccw
  line L402 (-247.4448, 62.5518) -> (-247.3498, 62.5518)
  line L403 (-247.3498, 62.5518) -> (-247.3448, 62.5518)
  line L404 (-246.7748, 62.5518) -> (-247.3448, 62.5518)
  line L405 (-246.7748, 62.5518) -> (-246.6798, 62.5518)
  line L406 (-246.6798, 62.5518) -> (-246.6748, 62.5518)
  arc A103 (-246.6748, 62.5518) -> (-246.4248, 62.5622) centre (-246.6748, 65.5518) ccw
  arc A104 (-246.4248, 62.5622) -> (-246.1748, 62.5518) centre (-246.1748, 65.5518) ccw
  line L407 (-246.1748, 62.5518) -> (-246.0798, 62.5518)
  line L408 (-246.0798, 62.5518) -> (-246.0748, 62.5518)
  line L409 (-245.5048, 62.5518) -> (-246.0748, 62.5518)
  line L410 (-245.5048, 62.5518) -> (-245.4098, 62.5518)
  line L411 (-245.4098, 62.5518) -> (-245.4048, 62.5518)
  arc A105 (-245.4048, 62.5518) -> (-245.1548, 62.5622) centre (-245.4048, 65.5518) ccw
  arc A106 (-245.1548, 62.5622) -> (-244.9048, 62.5518) centre (-244.9048, 65.5518) ccw
  line L412 (-244.9048, 62.5518) -> (-244.8098, 62.5518)
  line L413 (-244.8098, 62.5518) -> (-244.8048, 62.5518)
  line L414 (-244.2348, 62.5518) -> (-244.8048, 62.5518)
  line L415 (-244.2348, 62.5518) -> (-244.1398, 62.5518)
  line L416 (-244.1398, 62.5518) -> (-244.1348, 62.5518)
  arc A107 (-244.1348, 62.5518) -> (-243.8848, 62.5622) centre (-244.1348, 65.5518) ccw
  arc A108 (-243.8848, 62.5622) -> (-243.6348, 62.5518) centre (-243.6348, 65.5518) ccw
  line L417 (-243.6348, 62.5518) -> (-243.5398, 62.5518)
  line L418 (-243.5398, 62.5518) -> (-243.5348, 62.5518)
  line L419 (-242.9648, 62.5518) -> (-243.5348, 62.5518)
  line L420 (-242.9648, 62.5518) -> (-242.8698, 62.5518)
  line L421 (-242.8698, 62.5518) -> (-242.8648, 62.5518)
  arc A109 (-242.8648, 62.5518) -> (-242.6148, 62.5622) centre (-242.8648, 65.5518) ccw
  arc A110 (-242.6148, 62.5622) -> (-242.3648, 62.5518) centre (-242.3648, 65.5518) ccw
  line L422 (-242.3648, 62.5518) -> (-242.2698, 62.5518)
  line L423 (-242.2698, 62.5518) -> (-242.2648, 62.5518)
  line L424 (-241.6948, 62.5518) -> (-242.2648, 62.5518)
  line L425 (-241.6948, 62.5518) -> (-241.5998, 62.5518)
  line L426 (-241.5998, 62.5518) -> (-241.5948, 62.5518)
  arc A111 (-241.5948, 62.5518) -> (-241.3448, 62.5622) centre (-241.5948, 65.5518) ccw
  arc A112 (-241.3448, 62.5622) -> (-241.0948, 62.5518) centre (-241.0948, 65.5518) ccw
  line L427 (-241.0948, 62.5518) -> (-240.9998, 62.5518)
  line L428 (-240.9998, 62.5518) -> (-240.9948, 62.5518)
  line L429 (-240.4248, 62.5518) -> (-240.9948, 62.5518)
  line L430 (-240.4248, 62.5518) -> (-240.3298, 62.5518)
  line L431 (-240.3298, 62.5518) -> (-240.3248, 62.5518)
  arc A113 (-240.3248, 62.5518) -> (-240.0748, 62.5622) centre (-240.3248, 65.5518) ccw
  arc A114 (-240.0748, 62.5622) -> (-239.8248, 62.5518) centre (-239.8248, 65.5518) ccw
  line L432 (-239.8248, 62.5518) -> (-239.7298, 62.5518)
  line L433 (-239.7298, 62.5518) -> (-239.7248, 62.5518)
  line L434 (-239.1548, 62.5518) -> (-239.7248, 62.5518)
  line L435 (-239.1548, 62.5518) -> (-239.0598, 62.5518)
  line L436 (-239.0598, 62.5518) -> (-239.0548, 62.5518)
  arc A115 (-239.0548, 62.5518) -> (-238.8048, 62.5622) centre (-239.0548, 65.5518) ccw
  arc A116 (-238.8048, 62.5622) -> (-238.5548, 62.5518) centre (-238.5548, 65.5518) ccw
  line L437 (-238.5548, 62.5518) -> (-238.4598, 62.5518)
  line L438 (-238.4598, 62.5518) -> (-238.4548, 62.5518)
  line L439 (-237.8848, 62.5518) -> (-238.4548, 62.5518)
  line L440 (-237.8848, 62.5518) -> (-237.7898, 62.5518)
  line L441 (-237.7898, 62.5518) -> (-237.7848, 62.5518)
  arc A117 (-237.7848, 62.5518) -> (-237.5348, 62.5622) centre (-237.7848, 65.5518) ccw
  arc A118 (-237.5348, 62.5622) -> (-237.2848, 62.5518) centre (-237.2848, 65.5518) ccw
  line L442 (-237.2848, 62.5518) -> (-237.1898, 62.5518)
  line L443 (-237.1898, 62.5518) -> (-237.1848, 62.5518)
  line L444 (-236.6148, 62.5518) -> (-237.1848, 62.5518)
  line L445 (-236.6148, 62.5518) -> (-236.5198, 62.5518)
  line L446 (-236.5198, 62.5518) -> (-236.5148, 62.5518)
  arc A119 (-236.5148, 62.5518) -> (-236.2648, 62.5622) centre (-236.5148, 65.5518) ccw
  arc A120 (-236.2648, 62.5622) -> (-236.0148, 62.5518) centre (-236.0148, 65.5518) ccw
  line L447 (-236.0148, 62.5518) -> (-235.9198, 62.5518)
  line L448 (-235.9198, 62.5518) -> (-235.9148, 62.5518)
  line L449 (-235.3448, 62.5518) -> (-235.9148, 62.5518)
  line L450 (-235.3448, 62.5518) -> (-235.2498, 62.5518)
  line L451 (-235.2498, 62.5518) -> (-235.2448, 62.5518)
  arc A121 (-235.2448, 62.5518) -> (-234.9948, 62.5622) centre (-235.2448, 65.5518) ccw
  arc A122 (-234.9948, 62.5622) -> (-234.7448, 62.5518) centre (-234.7448, 65.5518) ccw
  line L452 (-234.7448, 62.5518) -> (-234.6498, 62.5518)
  line L453 (-234.6498, 62.5518) -> (-234.6448, 62.5518)
  line L454 (-234.0748, 62.5518) -> (-234.6448, 62.5518)
  line L455 (-234.0748, 62.5518) -> (-233.9798, 62.5518)
  line L456 (-233.9798, 62.5518) -> (-233.9748, 62.5518)
  arc A123 (-233.9748, 62.5518) -> (-233.7248, 62.5622) centre (-233.9748, 65.5518) ccw
  arc A124 (-233.7248, 62.5622) -> (-233.4748, 62.5518) centre (-233.4748, 65.5518) ccw
  line L457 (-233.4748, 62.5518) -> (-233.3798, 62.5518)
  line L458 (-233.3798, 62.5518) -> (-233.3748, 62.5518)
  line L459 (-232.8048, 62.5518) -> (-233.3748, 62.5518)
  line L460 (-232.8048, 62.5518) -> (-232.7098, 62.5518)
  line L461 (-232.7098, 62.5518) -> (-232.7048, 62.5518)
  arc A125 (-232.7048, 62.5518) -> (-232.4548, 62.5622) centre (-232.7048, 65.5518) ccw
  arc A126 (-232.4548, 62.5622) -> (-232.2048, 62.5518) centre (-232.2048, 65.5518) ccw
  line L462 (-232.2048, 62.5518) -> (-232.1098, 62.5518)
  line L463 (-221.9198, 62.5518) -> (-199.377, 62.5518)
  line L464 (-199.377, 62.5518) -> (-199.377, 86.5518)
  line L465 (-199.377, 86.5518) -> (-221.9198, 86.5518)
  arc A127 (-253.4198, 63.5518) -> (-252.4198, 62.5518) centre (-252.4198, 63.5518) ccw
  arc A128 (-252.4198, 86.5518) -> (-253.4198, 85.5518) centre (-252.4198, 85.5518) ccw
  dimension "d81" = 10
  dimension "d82" = 6
  dimension "d83" = 12
  dimension "d84" = 22
  dimension "d85" = 6
  dimension "d86" = 6
  dimension "d88" = 1
  constraint horizontal L60
  constraint vertical L61
  constraint horizontal L62
  constraint vertical L63
  constraint horizontal L64
  constraint vertical L65
  constraint horizontal L66
  constraint vertical L67
  constraint concentric A8 A10
  constraint concentric A9 A11
  constraint horizontal L463
  constraint vertical L464
  constraint horizontal L465
  constraint coincident L0 L464.end
  constraint coincident A50.end L264.end
  constraint coincident L263.start A50.start
  constraint coincident A49.end L259.end
  constraint coincident L258.start A49.start
  constraint coincident A48.end L254.end
  constraint coincident L253.start A48.start
  constraint coincident A47.end L249.end
  constraint coincident L248.start A47.start
  constraint coincident A46.end L244.end
  constraint coincident L243.start A46.start
  constraint coincident A45.end L239.end
  constraint coincident L238.start A45.start
  constraint coincident A44.end L234.end
  constraint coincident L233.start A44.start
  constraint coincident A43.end L227.end
  constraint coincident L226.start A42.start
  constraint coincident A41.end L220.end
  constraint coincident L219.start A41.start
  constraint coincident A40.end L215.end
  constraint coincident L214.start A40.start
  constraint coincident A39.end L210.end
  constraint coincident L209.start A39.start
  constraint coincident A38.end L205.end
  constraint coincident L204.start A38.start
  constraint coincident A37.end L200.end
  constraint coincident L199.start A37.start
  constraint coincident A36.end L195.end
  constraint coincident L194.start A36.start
  constraint coincident A35.end L189.end
  constraint coincident L188.start A35.start
  constraint coincident A34.end L184.end
  constraint coincident L183.start A34.start
  constraint coincident A33.end L179.end
  constraint coincident L178.start A33.start
  constraint coincident A32.end L174.end
  constraint coincident L173.start A32.start
  constraint coincident A31.end L169.end
  constraint coincident L168.start A31.start
  constraint coincident A30.end L164.end
  constraint coincident L163.start A30.start
  constraint coincident A29.end L159.end
  constraint coincident L158.start A29.start
  constraint coincident A28.end L154.end
  constraint coincident L153.start A28.start
  constraint coincident A27.end L149.end
  constraint coincident L148.start A27.start
  constraint coincident A26.end L144.end
  constraint coincident L143.start A26.start
  constraint coincident A25.end L138.end
  constraint coincident L137.start A25.start
  constraint coincident A24.end L133.end
  constraint coincident L132.start A24.start
  constraint coincident A23.end L128.end
  constraint coincident L127.start A23.start
  constraint coincident A22.end L123.end
  constraint coincident L122.start A22.start
  constraint coincident A21.end L118.end
  constraint coincident L117.start A21.start
  constraint coincident A20.end L113.end
  constraint coincident L112.start A20.start
  constraint coincident A19.end L108.end
  constraint coincident L107.start A19.start
  constraint coincident A18.end L103.end
  constraint coincident L102.start A18.start
  constraint coincident A17.end L98.end
  constraint coincident L97.start A17.start
  constraint coincident A16.end L93.end
  constraint coincident L92.start A16.start
  constraint coincident A15.end L88.end
  constraint coincident L87.start A15.start
  constraint coincident A14.end L83.end
  constraint coincident L82.start A14.start
  constraint coincident A13.end L78.end
  constraint coincident L77.start A13.start
  constraint coincident A12.end L73.end
  constraint coincident L72.start A12.start
  constraint tangent A100 L397
  constraint tangent L270 A51
  constraint tangent A52 L271
  constraint tangent A90 L371
  constraint tangent L275 A53
  constraint tangent L280 A55
  constraint tangent L285 A57
  constraint tangent A58 L286
  constraint tangent L295 A61
  constraint tangent L290 A59
  constraint tangent L300 A63
  constraint tangent A112 L427
  constraint tangent A64 L301
  constraint tangent A86 L361
  constraint tangent L355 A83
  constraint tangent L307 A65
  constraint tangent A66 L308
  constraint tangent L314 A67
  constraint tangent L319 A69
  constraint tangent A70 L320
  constraint tangent L334 A75
  constraint tangent L324 A71
  constraint tangent L329 A73
  constraint tangent L385 A95
  constraint tangent A126 L462
  constraint tangent A106 L412
  constraint tangent A84 L356
  constraint tangent A76 L335
  constraint tangent A94 L381
  constraint tangent L339 A77
  constraint tangent L345 A79
  constraint tangent L446 A119
  constraint tangent A80 L346
  constraint tangent L370 A89
  constraint tangent L350 A81
  constraint tangent A82 L351
  constraint tangent A110 L422
  constraint tangent A120 L447
  constraint tangent L360 A85
  constraint tangent L365 A87
  constraint tangent A88 L366
  constraint tangent L375 A91
  constraint tangent A118 L442
  constraint tangent A92 L376
  constraint tangent L380 A93
  constraint tangent A96 L386
  constraint tangent L390 A97
  constraint tangent A98 L391
  constraint tangent L396 A99
  constraint tangent L401 A101
  constraint tangent A102 L402
  constraint tangent L406 A103
  constraint tangent A104 L407
  constraint tangent L411 A105
  constraint tangent L416 A107
  constraint tangent A108 L417
  constraint tangent L421 A109
  constraint tangent L426 A111
  constraint tangent L431 A113
  constraint tangent A114 L432
  constraint tangent L436 A115
  constraint tangent A116 L437
  constraint tangent L441 A117
  constraint tangent L451 A121
  constraint tangent A122 L452
  constraint tangent L456 A123
  constraint tangent A124 L457
  constraint tangent L461 A125
  constraint tangent L393 A127
  constraint tangent L394 A127
  constraint tangent L342 A128
  constraint tangent L343 A128
  constraint equal A127 A128
  measures "d81" distance of L60.start L60.end
  measures "d82" distance of L60.start L62.end
  measures "d83" distance of L64.start L64.end
  measures "d84" distance of L64.start L66.end
  measures "d85" diameter of A10
  measures "d86" diameter of A11
  measures "d88" radius of A127
extrude "Extrude1" add sketch "Sketch1" along normal blind 2 contours L0 L1 L2 L3 L64 L65 L67 L266 L267 L268 L269 L270 A51 A52 L271 L272 L273 L274 L275 A53 A54 L276 L277 L278 L279 L280 A55 A56 L281 L282 L283 L284 L285 A57 A58 L286 L287 L288 L289 L290 A59 A60 L291 L292 L293 L294 L295 A61 A62 L296 L297 L298 L299 L300 A63 A64 L301 L302 L303 L304 L305 L306 L307 A65 A66 L308 L309 L310 L311 L312 L313 L314 A67 A68 L315 L316 L317 L318 L319 A69 A70 L320 L321 L322 L323 L324 A71 A72 L325 L326 L327 L328 L329 A73 A74 L330 L331 L332 L333 L334 A75 A76 L335 L336 L337 L338 L339 A77 A78 L340 L341 L342 L343 L344 L345 A79 A80 L346 L347 L348 L349 L350 A81 A82 L351 L352 L353 L354 L355 A83 A84 L356 L357 L358 L359 L360 A85 A86 L361 L362 L363 L364 L365 A87 A88 L366 L367 L368 L369 L370 A89 A90 L371 L372 L373 L374 L375 A91 A92 L376 L377 L378 L379 L380 A93 A94 L381 L382 L383 L384 L385 A95 A96 L386 L387 L388 L389 L390 A97 A98 L391 L392 L393 L394 L395 L396 A99 A100 L397 L398 L399 L400 L401 A101 A102 L402 L403 L404 L405 L406 A103 A104 L407 L408 L409 A124 L457 L458 L459 L460 L461 A125 A126 L462 L463 L465 A127 A128